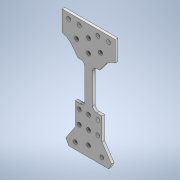
# Autodesk Inventor part: body_bone_4
Saved by Autodesk Inventor 2020 (Build 240168000, 168)
## iProperties
Created: 2019-05-16
Part Number: body_bone_4
Material: Generic
Document SubType Name: Modeling
Designer: psrob
Density: 1 g/cm^3
Appearance: Default
Author: psrob
Autodesk Inventor part; units mm, degrees
ref_plane "YZ Plane" through (0, 0, 0) normal (1, 0, 0) x (0, 1, 0)
ref_plane "XZ Plane" through (0, 0, 0) normal (0, 1, 0) x (-1, 0, 0)
ref_plane "XY Plane" through (0, 0, 0) normal (0, 0, 1) x (1, 0, 0)
sketch "Sketch1" plane through (0, 0, 0) normal (0, 0, 1) x (1, 0, 0)
  circle A0 centre (-14, 4) radius 1.5 projected
  circle A1 centre (-10, 13) radius 1.5 projected
  circle A2 centre (-7, 4) radius 1.5 projected
  line L0 (-20, 0) -> (-20, 8) projected
  line L1 (0, 0) -> (-20, 0) projected
  line L2 (0, 40) -> (0, 0) projected
  line L3 (-10, 40) -> (0, 40) projected
  line L4 (-10, 23) -> (-10, 40) projected
  line L5 (-10, 23) -> (-20, 8) projected
  circle A3 centre (14, 4) radius 1.5 projected
  circle A4 centre (10, 13) radius 1.5 projected
  circle A5 centre (7, 4) radius 1.5 projected
  line L6 (20, 0) -> (20, 8) projected
  line L7 (10, 23) -> (20, 8) projected
  line L8 (10, 23) -> (10, 40) projected
  line L9 (10, 40) -> (0, 40) projected
  line L10 (0, 40) -> (0, 0) projected
  line L11 (0, 0) -> (20, 0) projected
  line L12 (3, 84.8834) -> (-3, 84.8834) projected
  line L13 (-3, 84.8834) -> (-3, -165.1166) projected
  line L14 (3, -165.1166) -> (-3, -165.1166) projected
  line L15 (3, 84.8834) -> (3, -165.1166) projected
  circle A6 centre (-9, 80.8834) radius 1.5 projected
  circle A7 centre (-7, 90.8834) radius 1.5 projected
  circle A8 centre (-15, 90.8834) radius 1.5 projected
  line L16 (-12.05, 74.2834) -> (-8.0217, 68.9123) projected
  line L17 (-8.0217, 68.9123) -> (0, 68.9123) projected
  line L18 (0, 94.8834) -> (0, 68.9123) projected
  line L19 (0, 94.8834) -> (-20, 94.8834) projected
  line L20 (-20, 79.501) -> (-20, 94.8834) projected
  arc A9 (-12.05, 74.2834) -> (-20, 79.501) centre (-23.25, 65.8834) ccw projected
  line L21 (3, 94.8834) -> (3, 68.9123) projected
  circle A10 centre (9, 80.8834) radius 1.5 projected
  circle A11 centre (7, 90.8834) radius 1.5 projected
  circle A12 centre (15, 90.8834) radius 1.5 projected
  line L22 (12.05, 74.2834) -> (8.0217, 68.9123) projected
  arc A13 (20, 79.501) -> (12.05, 74.2834) centre (23.25, 65.8834) ccw projected
  line L23 (20, 79.501) -> (20, 94.8834) projected
  line L24 (0, 94.8834) -> (20, 94.8834) projected
  line L25 (0, 94.8834) -> (0, 68.9123) projected
  line L26 (8.0217, 68.9123) -> (0, 68.9123) projected
  line L27 (-20, 8) -> (20, 8)
  line L28 (-3, 40) -> (3, 40)
  line L29 (3, 40) -> (3, 68.9123)
  line L30 (3, 68.9123) -> (-3, 68.9123)
  line L31 (-3, 68.9123) -> (-3, 40)
  point P0 (3, 40)
  point P1 (-3, 68.9123)
  constraints: 10 end point, 2 parallel, 2 perpendicular, 2 point on line, 1 horizontal
extrude "Extrusion1" add sketch "Sketch1" along normal blind 2 contours L5 L4 L3 L13 L27 | L13 L3 L2 L27 | L13 L17 L26 L15 L9 L3 | L2 L9 L15 L27 | L17 L16 A9 L20 L19 L18 L12 L13 | L13 L12 L18 L17 | L15 L9 L8 L7 L27 | L18 L12 L15 L26 | L15 L21 L24 L23 A13 L22 L26 | L18 L24 L21 L12
chamfer "Chamfer1" distance 5 angle 45 2 edges at (20, 8, 1) (-20, 8, 1)
fillet "Fillet1" radius 3 4 edges at (3, 40, 1) (-3, 40, 1) (-3, 68.9123, 1) (3, 68.9123, 1)
sketch "Sketch2" plane through (0, 0, 2) normal (0, 0, 1) x (1, 0, 0)
  line L0 (-15, 8) -> (-17.2265, 12.1603) projected
  line L1 (-15, 8) -> (15, 8) projected
  line L2 (17.2265, 12.1603) -> (15, 8) projected
  line L3 (17.2265, 12.1603) -> (10, 23) projected
  line L4 (10, 23) -> (10, 40) projected
  line L5 (10, 40) -> (6, 40) projected
  arc A0 (3, 43) -> (6, 40) centre (6, 43) ccw projected
  line L6 (3, 43) -> (3, 65.9123) projected
  arc A1 (6, 68.9123) -> (3, 65.9123) centre (6, 65.9123) ccw projected
  line L7 (6, 68.9123) -> (8.0217, 68.9123) projected
  line L8 (8.0217, 68.9123) -> (12.05, 74.2834) projected
  arc A2 (20, 79.501) -> (12.05, 74.2834) centre (23.25, 65.8834) ccw projected
  line L9 (20, 79.501) -> (20, 94.8834) projected
  line L10 (20, 94.8834) -> (-20, 94.8834) projected
  line L11 (-20, 94.8834) -> (-20, 79.501) projected
  arc A3 (-12.05, 74.2834) -> (-20, 79.501) centre (-23.25, 65.8834) ccw projected
  line L12 (-12.05, 74.2834) -> (-8.0217, 68.9123) projected
  line L13 (-8.0217, 68.9123) -> (-6, 68.9123) projected
  arc A4 (-3, 65.9123) -> (-6, 68.9123) centre (-6, 65.9123) ccw projected
  line L14 (-3, 65.9123) -> (-3, 43) projected
  arc A5 (-6, 40) -> (-3, 43) centre (-6, 43) ccw projected
  line L15 (-6, 40) -> (-10, 40) projected
  line L16 (-10, 40) -> (-10, 23) projected
  line L17 (-10, 23) -> (-17.2265, 12.1603) projected
  circle A6 centre (10, 13) radius 1.5 projected
  circle A7 centre (7, 90.8834) radius 1.5 projected
  circle A8 centre (9, 80.8834) radius 1.5 projected
  circle A9 centre (15, 90.8834) radius 1.5 projected
  circle A10 centre (-9, 80.8834) radius 1.5 projected
  circle A11 centre (-7, 90.8834) radius 1.5 projected
  circle A12 centre (-15, 90.8834) radius 1.5 projected
  circle A13 centre (-10, 13) radius 1.5 projected
  circle A14 centre (7, 90.8834) radius 1.5 projected
  line L18 (7, 90.8834) -> (7, 35.8834)
  line L19 (7, 35.8834) -> (7, 25.8834)
  circle A15 centre (7, 35.8834) radius 1.5
  circle A16 centre (7, 25.8834) radius 1.5
  circle A17 centre (-7, 90.8834) radius 1.5 projected
  line L20 (-7, 90.8834) -> (-7, 35.8834)
  line L21 (-7, 35.8834) -> (-7, 25.8834)
  circle A18 centre (-7, 35.8834) radius 1.5
  circle A19 centre (-7, 25.8834) radius 1.5
  line L22 (-7, 35.8834) -> (7, 35.8834)
  line L23 (-7, 25.8834) -> (7, 25.8834)
  circle A20 centre (0, 35.8834) radius 1.5
  circle A21 centre (0, 25.8834) radius 1.5
  line L24 (0, 25.8834) -> (0, 15.8834)
  circle A22 centre (0, 15.8834) radius 1.5
  line L25 (0, 35.8834) -> (0, 75.8834)
  line L26 (0, 75.8834) -> (0, 85.8834)
  circle A23 centre (0, 85.8834) radius 1.5
  circle A24 centre (0, 75.8834) radius 1.5
  point P0 (0, 0)
  dimension "d6" = 55
  dimension "d7" = 10
  dimension "d8" = 3
  dimension "d9" = 3
  dimension "d10" = 55
  dimension "d11" = 10
  dimension "d12" = 3
  dimension "d13" = 3
  dimension "d14" = 3
  dimension "d15" = 3
  dimension "d16" = 10
  dimension "d17" = 3
  dimension "d18" = 40
  dimension "d19" = 10
  dimension "d20" = 3
  dimension "d21" = 3
  constraints: 18 end point, 9 centre point, 7 coincident, 3 point on line, 2 midpoint, 2 vertical, 1 parallel, 1 perpendicular
  measures "d6" distance of L18.start L18.end
  measures "d7" distance of L18.end L19.end
  measures "d8" diameter of A15
  measures "d9" diameter of A16
  measures "d10" distance of L20.start L20.end
  measures "d11" distance of L20.end L21.end
  measures "d12" diameter of A18
  measures "d13" diameter of A19
  measures "d14" diameter of A20
  measures "d15" diameter of A21
  measures "d16" distance of L24.start L24.end
  measures "d17" diameter of A22
  measures "d18" distance of L25.start L25.end
  measures "d19" distance of L25.end L26.end
  measures "d20" diameter of A23
  measures "d21" diameter of A24
extrude "Extrusion2" cut sketch "Sketch2" against normal blind 10 contours A22 | A23 | A24 L26 L25 | L25 L26 A24 | A18 L22 L20 | L20 L21 A18 | L22 A18 L21 | A15 L19 L18 | L18 L22 A15 | A20 L25 L22 | L22 A20 | A19 L23 L21 | L21 L23 A19 | L19 A15 L22 | L25 A20 L22 | A21 L23 | L23 L24 A21 | A16 L23 L19 | L19 L23 A16 | L23 A21 L24
body "Solid1"
